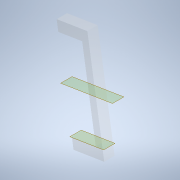
# Autodesk Inventor part: arm
Saved by Autodesk Inventor 2021 (Build 250183000, 183)
## iProperties
Created: 2022-05-21
Part Number: arm
Material: PET Plastic
Document SubType Name: Modeling
Designer: techv
Mass: 442.753 g
Surface Area: 446.747 cm^2
Volume: 287.315 cm^3
Density: 1.541 g/cm^3
Appearance: Polycarbonate - Clear
Author: techv
Autodesk Inventor part; units mm, degrees
ref_plane "YZ Plane" through (0, 0, 0) normal (1, 0, 0) x (0, 1, 0)
ref_plane "XZ Plane" through (0, 0, 0) normal (0, 1, 0) x (-1, 0, 0)
ref_plane "XY Plane" through (0, 0, 0) normal (0, 0, 1) x (1, 0, 0)
sketch "Sketch1" plane through (0, 0, 0) normal (0, 0, 1) x (1, 0, 0)
  arc A0 (5.5018, -3.1706) -> (4.1426, 4.8126) centre (0, 0) ccw projected
  line L0 (-0.2789, 17.1872) -> (4.1426, 4.8126) projected
  arc A1 (-0.2789, 17.1872) -> (-5.4243, 16.3111) centre (-2.7743, 16.2955) ccw projected
  line L1 (-5.5018, 3.1706) -> (-5.4243, 16.3111) projected
  arc A2 (-5.5018, 3.1706) -> (-4.1426, -4.8126) centre (0, 0) ccw projected
  line L2 (-4.1426, -4.8126) -> (0.2789, -17.1872) projected
  arc A3 (0.2789, -17.1872) -> (5.4243, -16.3111) centre (2.7743, -16.2955) ccw projected
  line L3 (5.4243, -16.3111) -> (5.5018, -3.1706) projected
  circle A4 centre (1.7673, -10.3806) radius 0.5 projected
  circle A5 centre (1.2638, -7.4232) radius 0.5 projected
  circle A6 centre (0, 0) radius 4.375 projected
  circle A7 centre (-2.2708, 13.3381) radius 0.5 projected
  circle A8 centre (-1.7673, 10.3806) radius 0.5 projected
  circle A9 centre (-1.2638, 7.4232) radius 0.5 projected
  circle A10 centre (-2.7743, 16.2955) radius 0.5 projected
  circle A11 centre (2.2708, -13.3381) radius 0.5 projected
  circle A12 centre (2.7743, -16.2955) radius 0.5 projected
  line L4 (0, 0) -> (2.7743, -16.2955)
  line L5 (0, 0) -> (47.7501, -296.1755)
  line L6 (0, 0) -> (23.8751, -148.0877)
  line L7 (-9.8725, -1.5917) -> (37.8776, -297.7672)
  line L8 (37.8776, -297.7672) -> (57.6226, -294.5838)
  line L9 (57.6226, -294.5838) -> (9.8725, 1.5917)
  line L10 (9.8725, 1.5917) -> (-9.8725, -1.5917)
  line L11 (-9.8725, -1.5917) -> (57.6226, -294.5838) construction
  line L12 (37.8776, -297.7672) -> (9.8725, 1.5917) construction
  circle A13 centre (0, 0) radius 25
  point P0 (13.5195, -21.0291)
  point P1 (-6.2255, -24.2124)
  dimension "d0" = 300
  dimension "d1" = 150
  dimension "d2" = 20
  dimension "d3" = 50
  constraints: 18 end point, 3 midpoint, 2 parallel, 1 centre point, 1 coincident, 1 perpendicular
  measures "d0" distance of L4.start L5.end
  measures "d1" distance of L4.start L6.end
  measures "d2" distance of L8.end L7.end
  measures "d3" diameter of A13
extrude "Extrusion1" add sketch "Sketch1" along normal blind 30 contours L3 A3 L5 A12 L4 A11 A4 A5 A6 L10 A0 | A0 L10 L9 A13 L5 A3 L3 | L10 A6 A2 L1 A1 L0 A0 | A0 L0 A1 L1 A2 L10 L7 A13 L9 | L10 A6 | A6 L4 L10 | L5 A13 L7 L10 A2 L2 A3 | A3 L2 A2 L10 A6 L5 A5 A4 A11 A12 | L9 L8 L5 A13 | L10 L5 A6 | L4 A6 L5 | L5 A12 | A12 L5 | L5 L8 L7 A13 | L4 A5 L5 A6 | L5 A11 L4 A12 | L4 A5 L5 | A5 L4 | L5 A5 | L5 A11 L4 | A11 L5 | L4 A4 L5 A5 | L4 A11 | L5 A4 L4 A11 | L4 A4 L5 | A4 L4 | L5 A4 | A7 | A8 | A9 | A10
sketch "Sketch2" plane through (37.8776, -297.7672, 0) normal (-0.9872517, -0.159167, 0) x (0, 0, 1)
  line L0 (30, 277.0871) -> (30, 0) projected
  line L1 (30, 0) -> (0, 0)
  line L2 (0, 0) -> (0, 30)
  line L3 (0, 30) -> (30, 30)
  line L4 (30, 30) -> (30, 0)
  point P0 (0, 300)
  point P1 (30, 30)
  dimension "d6" = 30
  dimension "d7" = 30
  constraints: 8 end point, 2 parallel, 1 horizontal, 1 perpendicular
  measures "d6" distance of L2.end L3.end
  measures "d7" distance of L1.end L2.end
extrude "Extrusion2" add sketch "Sketch2" along normal blind 70
sketch "Sketch4" plane through (0, 0, 30) normal (0, 0, 1) x (1, 0, 0)
  line L0 (-6.2255, -24.2124) -> (33.1026, -268.1496) projected
  line L1 (33.1026, -268.1496) -> (-36.005, -279.2913) projected
  line L2 (-31.23, -308.9089) -> (-36.005, -279.2913) projected
  line L3 (57.6226, -294.5838) -> (-31.23, -308.9089) projected
  line L4 (57.6226, -294.5838) -> (13.5195, -21.0291) projected
  arc A0 (13.5195, -21.0291) -> (-6.2255, -24.2124) centre (0, 0) ccw projected
  arc A1 (13.5195, -21.0291) -> (-6.2255, -24.2124) centre (0, 0) ccw projected
  circle A2 centre (0, 0) radius 25
  point P0 (13.5195, -21.0291)
  constraints: 1 centre point, 1 coincident
extrude "Extrusion4" cut sketch "Sketch4" against normal through all contours A0 A2
sketch "Sketch5" plane through (0, 0, 30) normal (0, 0, 1) x (1, 0, 0)
  arc A0 (-6.2255, -24.2124) -> (13.5195, -21.0291) centre (0, 0) ccw projected
  line L0 (-6.2255, -24.2124) -> (33.1026, -268.1496) projected
  line L1 (33.1026, -268.1496) -> (-36.005, -279.2913) projected
  line L2 (-31.23, -308.9089) -> (-36.005, -279.2913) projected
  line L3 (57.6226, -294.5838) -> (-31.23, -308.9089) projected
  line L4 (57.6226, -294.5838) -> (13.5195, -21.0291) projected
  line L5 (-6.2255, -24.2124) -> (33.1026, -268.1496) projected
  line L6 (-6.2255, -24.2124) -> (13.5195, -21.0291)
  constraints: 2 end point, 1 perpendicular
extrude "Extrusion5" add sketch "Sketch5" against normal up to surface (30 mm away) contours L6 A0
ref_plane "Work Plane2" through (33.1836, -142.9977, 0) normal (0.159167, -0.9872517, 0) x (0.9872517, 0.159167, 0)
ref_plane "Work Plane1" through (52.8476, -264.9663, 0) normal (0.159167, -0.9872517, 0) x (0.9872517, 0.159167, 0)
mirror "Mirror1" about plane through (33.1836, -142.9977, 0) normal (0.159167, -0.9872517, 0) of "Extrusion2"
mirror "Mirror2" about plane through (33.1836, -142.9977, 0) normal (0.159167, -0.9872517, 0) of "Extrusion1"
sketch "Sketch6" plane through (0, 0, 30) normal (0, 0, 1) x (1, 0, 0)
  line L0 (33.1026, -268.1496) -> (-36.005, -279.2913) projected
  line L1 (-31.23, -308.9089) -> (-36.005, -279.2913) projected
  line L2 (24.0813, -299.9914) -> (-31.23, -308.9089) projected
  arc A0 (24.0813, -299.9914) -> (52.8476, -264.9663) centre (46.6221, -289.1787) ccw projected
  line L3 (52.8476, -264.9663) -> (8.7445, 8.5884) projected
  line L4 (-80.1082, -5.7366) -> (8.7445, 8.5884) projected
  line L5 (-80.1082, -5.7366) -> (-75.3332, -35.3541) projected
  line L6 (-6.2255, -24.2124) -> (-75.3332, -35.3541) projected
  line L7 (-6.2255, -24.2124) -> (33.1026, -268.1496) projected
  line L8 (-36.005, -279.2913) -> (-31.23, -308.9089) projected
  line L9 (-36.005, -279.2913) -> (52.8476, -264.9663)
  line L10 (24.0813, -299.9914) -> (-31.23, -308.9089) projected
  line L11 (-31.23, -308.9089) -> (57.6226, -294.5838)
  line L12 (57.6226, -294.5838) -> (52.8476, -264.9663)
  point P0 (0, 0)
  constraints: 6 end point, 2 perpendicular, 1 collinear
extrude "Extrusion6" cut sketch "Sketch6" against normal through all contours A0 L11 L12
sketch "Sketch7" plane through (0, 0, 30) normal (0, 0, 1) x (1, 0, 0)
  point P0 (0, 0)
sketch "Sketch8" plane through (0, 0, 30) normal (0, 0, 1) x (1, 0, 0)
  line L0 (-31.23, -308.9089) -> (-36.005, -279.2913) projected
  line L1 (-6.2255, -24.2124) -> (33.1026, -268.1496) projected
  line L2 (-36.005, -279.2913) -> (33.1026, -268.1496)
  point P0 (0, 0)
  constraints: 2 end point, 1 perpendicular
body "Solid1"
